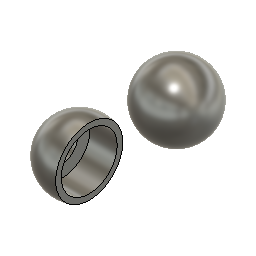
eyes (Autodesk Fusion 360 design; units mm, degrees)
part number: 2026-08-12-21-56-08-420
Autodesk Fusion 360 part; units mm, degrees
sketch "Sketch1" plane through (0, 0, 0) normal (1, 0, 0) x (0, 0, -1)
  circle A0 centre (30, 30) radius 9
  circle A1 centre (30, 30) radius 6
  circle A2 centre (30, 30) radius 4
  dimension "d1" = 18
  dimension "d2" = 12
  dimension "d7" = 8
  constraint concentric A0 A1
  constraint concentric A1 A2
  measures "d1" diameter of A0
  measures "d2" diameter of A1
  measures "d7" diameter of A2
sketch "Sketch2" plane through (0, 0, 0) normal (1, 0, 0) x (0, 0, -1)
  circle A0 centre (30, 30) radius 7.2
  circle A1 centre (30, 30) radius 8.2
  dimension "d3" = 14.4
  dimension "d5" = 16.4
  constraint concentric A0 A1
  measures "d3" diameter of A0
  measures "d5" diameter of A1
sphere "SpherePrimitive1" add diameter 18 placed x (0, 0, -1) y (0, 1, 0) z (1, 0, 0) at (0, 30, -30) makes body 1
extrude "Extrude1" cut sketch "Sketch1" against normal blind 2 from surface at -8 contours A2 bodies 1
extrude "Extrude3" cut sketch "Sketch2" along normal blind 18 from surface at -4.5 contours A0 bodies 1
extrude "Extrude4" cut sketch "Sketch2" along normal blind 5 from surface at 2.5 contours A0 | A1 bodies 1
extrude "Extrude5" cut 1 faces at (-8, 28.3658, -29.213) along direction (1, 0, 0) blind 3.5 on bodies 1 bodies 1
extrude "Extrude6" cut sketch "Sketch1" along normal blind 2 from surface at 2.5 contours A0 | A1 | A2 bodies 1
sphere "SpherePrimitive2" add diameter 18 placed x (0, 0, -1) y (0, 1, 0) z (1, 0, 0) at (0, 30, -55) separate body makes body 2
named bodies: "camera eye", "eye"
